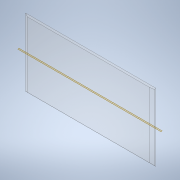
# Autodesk Inventor part: Wind Tunnel Test Section Back
Saved by Autodesk Inventor 2020 (Build 240168000, 168)
## iProperties
Created: 2022-03-06
Part Number: Wind Tunnel Test Section Back
Material: Polycarbonate, Clear
Document SubType Name: Modeling
Designer: kamer
Density: 1.2 g/cm^3
Appearance: Polycarbonate - Clear
Author: kamer
Autodesk Inventor part; units mm, degrees
ref_plane "YZ Plane" through (0, 0, 0) normal (1, 0, 0) x (0, 1, 0)
ref_plane "XY Plane" through (0, 0, 0) normal (0, 0, 1) x (1, 0, 0)
sketch "Sketch1" plane through (0, 0, 0) normal (0, 0, 1) x (1, 0, 0)
  line L0 (0, 0) -> (609.6, 0)
  line L1 (609.6, 0) -> (609.6, 317.881)
  line L2 (609.6, 317.881) -> (0, 317.881)
  line L3 (0, 317.881) -> (0, 0)
  dimension "d0" = 609.6
  dimension "d1" = 317.881
  constraints: 8 end point, 2 parallel, 1 horizontal, 1 perpendicular
  measures "d0" distance of L1.end L2.end
  measures "d1" distance of L0.end L1.end
extrude "Extrusion1" add sketch "Sketch1" along normal blind 5.7658
sketch "Sketch2" plane through (0, 317.881, 0) normal (0, 1, 0) x (1, 0, 0)
  line L0 (609.6, 0) -> (0, 0) projected
  line L1 (0, 0) -> (0, -5.7658) projected
  line L2 (609.6, -5.7658) -> (0, -5.7658) projected
  line L3 (609.6, 0) -> (609.6, -5.7658) projected
  line L4 (0, 0) -> (609.6, 0) projected
  line L5 (0, 0) -> (14.4594, -5.7658)
  line L6 (0, -5.7658) -> (609.6, -5.7658) projected
  line L7 (14.4594, -5.7658) -> (14.4594, 0)
  line L8 (14.4594, -5.7658) -> (20.2252, -5.7658) construction
  dimension "d4" = 21.74
  dimension "d5" = 90
  constraints: 6 end point, 2 point on line, 1 horizontal, 1 perpendicular
  measures "d4" angle of L5 L0
  measures "d5" angle of L8 L7
extrude "Extrusion2" cut sketch "Sketch2" against normal through all contours L5 L2 L1
sketch "Sketch3" plane through (609.6, 0, 0) normal (1, 0, 0) x (0, 0, -1)
  line L0 (0, 0) -> (0, 317.881) projected
  line L1 (0, 317.881) -> (-5.7658, 317.881) projected
  line L2 (-5.7658, 0) -> (-5.7658, 317.881) projected
  line L3 (0, 0) -> (-5.7658, 0) projected
  line L4 (0, 0) -> (-5.7658, 0) projected
  line L5 (0, 0) -> (-5.7658, 5.7658)
  line L6 (-5.7658, 0) -> (-5.7658, 317.881) projected
  line L7 (0, 0) -> (8.1541, 0) construction
  line L8 (0, 317.881) -> (-5.7658, 317.881) projected
  line L9 (0, 317.881) -> (-5.7658, 312.1152)
  line L10 (0, 317.881) -> (8.1541, 317.881) construction
  dimension "d8" = 135
  dimension "d9" = 135
  constraints: 8 end point, 2 equal length, 2 horizontal, 2 point on line
  measures "d8" angle of L7 L5
  measures "d9" angle of L9 L10
extrude "Extrusion3" cut sketch "Sketch3" against normal through all contours L3 L2 L5 | L9 L2 L1
ref_plane "Work Plane1" through (0, 158.9405, 0) normal (0, 1, 0) x (-1, 0, 0)
sketch "Sketch4" plane through (0, 158.9405, 0) normal (0, 1, 0) x (-1, 0, 0)
  line L0 (-14.4594, 5.7658) -> (0, 0) projected
  line L1 (-609.6, 5.7658) -> (-14.4594, 5.7658) projected
  line L2 (-609.6, 0) -> (-609.6, 5.7658) projected
  line L3 (-609.6, 0) -> (0, 0) projected
  line L4 (-609.6, 5.7658) -> (-584.2, 5.7658) construction
  line L5 (-584.2, 5.7658) -> (-609.6, 4.4413)
  point P0 (0, 0)
  dimension "d13" = 25.4
  dimension "d14" = 2.985
  constraints: 4 end point, 2 point on line
  measures "d13" distance of L1.start L4.end
  measures "d14" angle of L4 L5
extrude "Extrusion4" cut sketch "Sketch4" against normal through all both and the other way through all contours L5 L2 L1
body "Solid1"
